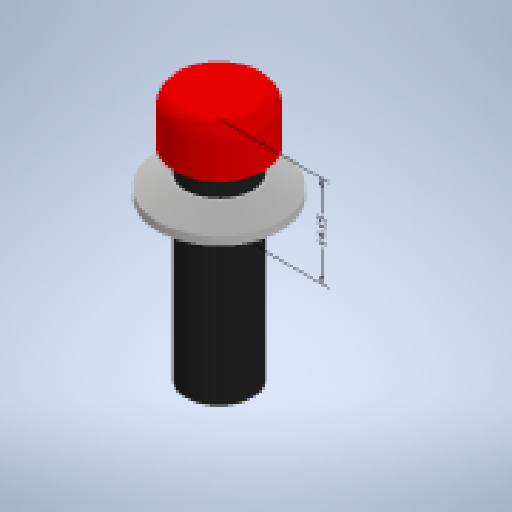
# Autodesk Inventor part: pannel_push_sw._redipt
Saved by Autodesk Inventor 2026.1 (Build 301233020, 233B)
## iProperties
Created: 2026-01-19
Part Number: pannel_push_sw._redipt
Material: 一般
Document SubType Name: Modeling
Designer: hibik
Density: 1 g/cm^3
Appearance: 既定
Author: hibik
Autodesk Inventor part; units mm, degrees
ref_plane "YZ Plane" through (0, 0, 0) normal (1, 0, 0) x (0, 1, 0)
ref_plane "XZ Plane" through (0, 0, 0) normal (0, 1, 0) x (-1, 0, 0)
ref_plane "XY Plane" through (0, 0, 0) normal (0, 0, 1) x (1, 0, 0)
sketch "スケッチ1" plane through (0, 0, 0) normal (0, 1, 0) x (-1, 0, 0)
  circle A0 centre (0, 0) radius 5.1
  dimension "d0" = 10.2
  constraints: 1 centre point, 1 coincident
  measures "d0" diameter of A0
extrude "押し出し1" add sketch "スケッチ1" along normal blind 24.5
sketch "スケッチ2" plane through (0, 24.5, 0) normal (0, 1, 0) x (1, 0, 0)
  circle A0 centre (0, 0) radius 9.47
  dimension "d3" = 18.94
  constraints: 1 centre point, 1 coincident
  measures "d3" diameter of A0
extrude "押し出し2" add sketch "スケッチ2" along normal blind 6.75
sketch "スケッチ3" plane through (0, 31.25, 0) normal (0, 1, 0) x (1, 0, 0)
  circle A0 centre (0, 0) radius 6.885
  dimension "d6" = 13.77
  constraints: 1 centre point, 1 coincident
  measures "d6" diameter of A0
extrude "押し出し3" add sketch "スケッチ3" along normal blind 7.4
sketch "スケッチ4" plane through (0, 31.25, 0) normal (0, 1, 0) x (1, 0, 0)
  circle A0 centre (0, 0) radius 9.47 projected
  circle A1 centre (0, 0) radius 5.1
  dimension "d9" = 10.2
  constraints: 1 centre point, 1 coincident
  measures "d9" diameter of A1
extrude "押し出し4" cut sketch "スケッチ4" against normal blind 3.5
chamfer "面取り1" distance 2 distance2 4 1 edges at (-9.47, 27.75, 0) measured on face at (9.4393, 26.6667, 0.762)
fillet "フィレット1" radius 2 1 edges at (-6.885, 38.65, 0)
